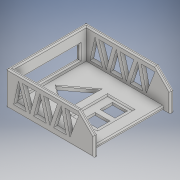
# Autodesk Inventor part: Base-Motherboard-v2
Saved by Autodesk Inventor 2018 (Build 220112000, 112)
## iProperties
Created: 2017-07-20
Part Number: Base-Motherboard-v2
Material: Generic
Document SubType Name: Modeling
Designer: JAck
Density: 1 g/cm^3
Appearance: Default
Author: JAck
Autodesk Inventor part; units mm, degrees
ref_plane "YZ Plane" through (0, 0, 0) normal (1, 0, 0) x (0, 1, 0)
ref_plane "XZ Plane" through (0, 0, 0) normal (0, 1, 0) x (-1, 0, 0)
ref_plane "XY Plane" through (0, 0, 0) normal (0, 0, 1) x (1, 0, 0)
sketch "Sketch1" plane through (0, 0, 0) normal (0, 1, 0) x (-1, 0, 0)
  line L0 (72.6415, 114.85) -> (-102.3585, 114.85)
  line L1 (-102.3585, 114.85) -> (-102.3585, -45.15)
  line L2 (-102.3585, -45.15) -> (72.6415, -45.15)
  line L3 (72.6415, -45.15) -> (72.6415, 114.85)
  line L4 (65.1415, 107.35) -> (-102.3585, 107.35)
  line L5 (-102.3585, 107.35) -> (-102.3585, -37.65)
  line L6 (-102.3585, -37.65) -> (65.1415, -37.65)
  line L7 (65.1415, -37.65) -> (65.1415, 107.35)
  line L8 (-102.3585, -37.65) -> (-89.8585, -37.65)
  line L9 (-89.8585, -37.65) -> (-89.8585, 107.35)
  line L10 (-89.8585, 107.35) -> (-102.3585, 107.35)
  line L11 (-102.3585, 107.35) -> (-102.3585, -37.65)
  point P0 (0, 0)
  dimension "d0" = 175
  dimension "d1" = 160
  dimension "d2" = 7.5
  dimension "d3" = 0
  dimension "d4" = 7.5
  dimension "d5" = 7.5
  dimension "d6" = 145
  dimension "d7" = 167.5
  dimension "d8" = 12.5
  constraints: 24 end point, 6 parallel, 3 horizontal, 3 perpendicular, 1 point on line
  measures "d0" distance between parallel lines of L1 L3
  measures "d1" distance of L0.end L1.end
  measures "d2" distance between parallel lines of L3 L7
  measures "d3" distance between parallel lines of L1 L5
  measures "d4" distance between parallel lines of L2 L6
  measures "d5" distance between parallel lines of L0 L4
  measures "d6" distance between parallel lines of L6 L4
  measures "d7" distance between parallel lines of L5 L7
  measures "d8" distance between parallel lines of L9 L1
extrude "Extrusion1" add sketch "Sketch1" along normal blind 60 contours L3 L2 L1 L6 L7 L4 L0
sketch "Sketch2" plane through (-72.6415, 0, -45.15) normal (-1, 0, 0) x (0, 0, 1)
  line L0 (20, 52.5) -> (140, 52.5)
  line L1 (140, 52.5) -> (140, 25)
  line L2 (140, 25) -> (20, 25)
  line L3 (20, 25) -> (20, 52.5)
  line L4 (160, 0) -> (160, 60) projected
  line L5 (0, 0) -> (0, 60) projected
  line L6 (0, 60) -> (160, 60) projected
  line L7 (0, 0) -> (160, 0) projected
  point P0 (45.15, 0)
  dimension "d11" = 20
  dimension "d12" = 20
  dimension "d13" = 7.5
  dimension "d14" = 25
  dimension "d15" = 120
  dimension "d16" = 27.5
  constraints: 8 end point, 2 parallel, 1 horizontal, 1 perpendicular
  measures "d11" distance between parallel lines of L4 L1
  measures "d12" distance between parallel lines of L5 L3
  measures "d13" distance between parallel lines of L6 L0
  measures "d14" distance between parallel lines of L7 L2
  measures "d15" distance between parallel lines of L3 L1
  measures "d16" distance of L0.end L1.end
extrude "Extrusion2" cut sketch "Sketch2" against normal blind 60 contours L0 L1 L2 L3
sketch "Sketch3" plane through (0, 60, 0) normal (0, 1, 0) x (1, 0, 0)
  line L0 (-72.6415, -114.85) -> (102.3585, -114.85) projected
  line L1 (102.3585, 45.15) -> (-72.6415, 45.15) projected
  line L2 (-72.6415, -114.85) -> (102.3585, -114.85)
  line L3 (102.3585, -114.85) -> (102.3585, 45.15)
  line L4 (102.3585, 45.15) -> (-72.6415, 45.15)
  line L5 (-72.6415, 45.15) -> (-72.6415, -114.85)
  point P0 (0, 0)
  constraints: 8 end point, 2 parallel, 1 horizontal, 1 perpendicular
extrude "Extrusion3" add sketch "Sketch3" along normal blind 7.5
sketch "Sketch4" plane through (0, 60, 0) normal (0, -1, 0) x (1, 0, 0)
  line L0 (-65.1415, 107.35) -> (102.3585, 107.35) projected
  line L1 (102.3585, -37.65) -> (-65.1415, -37.65) projected
  line L2 (102.3585, 107.35) -> (89.8585, 107.35)
  line L3 (89.8585, 107.35) -> (89.8585, -37.65)
  line L4 (89.8585, -37.65) -> (102.3585, -37.65)
  line L5 (102.3585, -37.65) -> (102.3585, 107.35)
  point P0 (0, 0)
  dimension "d21" = 12.5
  constraints: 8 end point, 2 parallel, 1 horizontal, 1 perpendicular, 1 point on line
  measures "d21" distance between parallel lines of L5 L3
extrude "Extrusion4" cut sketch "Sketch4" against normal blind 7.5
chamfer "Chamfer1" distance 30 angle 45 2 edges at (102.3585, 0, 111.1) (102.3585, 0, -41.4)
sketch "Sketch5" plane through (0, 67.5, 0) normal (0, 1, 0) x (1, 0, 0)
  line L0 (59.8585, -4.85) -> (29.8585, -4.85)
  line L1 (29.8585, -4.85) -> (29.8585, -29.85)
  line L2 (29.8585, -29.85) -> (59.8585, -29.85)
  line L3 (59.8585, -29.85) -> (59.8585, -4.85)
  line L4 (59.8585, -64.85) -> (29.8585, -64.85)
  line L5 (29.8585, -64.85) -> (29.8585, -39.85)
  line L6 (29.8585, -39.85) -> (59.8585, -39.85)
  line L7 (59.8585, -39.85) -> (59.8585, -64.85)
  line L8 (89.8585, -107.35) -> (89.8585, 37.65) projected
  line L9 (-72.6415, -114.85) -> (102.3585, -114.85) projected
  line L10 (102.3585, 45.15) -> (-72.6415, 45.15) projected
  point P0 (0, 0)
  dimension "d27" = 30
  dimension "d28" = 30
  dimension "d29" = 10
  dimension "d30" = 50
  dimension "d31" = 50
  dimension "d32" = 25
  dimension "d33" = 30
  dimension "d34" = 30
  constraints: 16 end point, 4 parallel, 2 horizontal, 2 perpendicular, 1 point on line
  measures "d27" distance between parallel lines of L8 L3
  measures "d28" distance between parallel lines of L8 L7
  measures "d29" distance between parallel lines of L6 L2
  measures "d30" distance between parallel lines of L9 L4
  measures "d31" distance between parallel lines of L10 L0
  measures "d32" distance of L0.end L1.end
  measures "d33" distance of L0.start L0.end
  measures "d34" distance between parallel lines of L7 L5
extrude "Extrusion5" cut sketch "Sketch5" against normal blind 7.5
sketch "Sketch6" plane through (0, 60, 0) normal (0, -1, 0) x (1, 0, 0)
  line L0 (64.8585, 69.85) -> (14.8585, 69.85)
  line L1 (14.8585, 69.85) -> (14.8585, -0.15)
  line L2 (14.8585, -0.15) -> (64.8585, -0.15)
  line L3 (64.8585, -0.15) -> (64.8585, 69.85)
  line L4 (59.8585, 64.85) -> (59.8585, 39.85) projected
  line L5 (29.8585, 39.85) -> (29.8585, 64.85) projected
  line L6 (29.8585, 64.85) -> (59.8585, 64.85) projected
  line L7 (59.8585, 4.85) -> (29.8585, 4.85) projected
  point P0 (0, 0)
  dimension "d37" = 5
  dimension "d38" = 15
  dimension "d39" = 5
  dimension "d40" = 5
  constraints: 8 end point, 2 parallel, 1 horizontal, 1 perpendicular
  measures "d37" distance between parallel lines of L3 L4
  measures "d38" distance between parallel lines of L5 L1
  measures "d39" distance between parallel lines of L6 L0
  measures "d40" distance between parallel lines of L2 L7
extrude "Extrusion6" cut sketch "Sketch6" against normal blind 2.5
fillet "Fillet1" radius 2.5 33 edges at (89.8585, 60, 34.85) (102.3585, 48.75, -45.15) (87.3585, 15, -45.15) (102.3585, 48.75, 107.35) (102.3585, 48.75, -37.65) (87.3585, 15, -37.65) (87.3585, 15, 107.35) (87.3585, 15, 114.85) (102.3585, 48.75, 114.85) (3.6085, 0, 107.35) (-0.1415, 0, 114.85) (-0.1415, 0, -45.15) (3.6085, 0, -37.65) (-72.6415, 0, 34.85) (-65.1415, 0, 34.85) (-72.6415, 52.5, 34.85) (-72.6415, 38.75, 94.85) (-72.6415, 25, 34.85) (-72.6415, 38.75, -25.15) (-65.1415, 52.5, 34.85) (-65.1415, 38.75, 94.85) (-65.1415, 25, 34.85) (-65.1415, 38.75, -25.15) (-72.6415, 33.75, 114.85) (-72.6415, 33.75, -45.15) (14.8585, 67.5, 114.85) (-72.6415, 67.5, 34.85) (14.8585, 67.5, -45.15) (89.8585, 67.5, 34.85) (14.8585, 60, 34.85) (39.8585, 60, 69.85) (64.8585, 60, 34.85) (39.8585, 60, -0.15)
sketch "Sketch9" plane through (99.8585, 65, -45.15) normal (0, 0, -1) x (-1, 0, 0)
  line L0 (165, -62.5) -> (165, -5) projected
  line L1 (165, -10) -> (0, -10)
  line L2 (0, 0) -> (0, -33.9645) projected
  line L3 (173.9645, -55) -> (21.0355, -55)
  line L4 (0, -33.9645) -> (28.5355, -62.5) projected
  line L5 (170, -62.5) -> (28.5355, -62.5) projected
  line L6 (0, 0) -> (170, 0) projected
  line L7 (157.5, -10) -> (147.5, -55)
  line L8 (147.5, -55) -> (132.5, -10)
  line L9 (125, -10) -> (140, -55)
  line L10 (125, -10) -> (112.5, -55)
  line L11 (105, -55) -> (117.5, -10)
  line L12 (105, -55) -> (92.5, -10)
  line L13 (97.5, -55) -> (85, -10)
  line L14 (85, -10) -> (70, -55)
  line L15 (62.5, -55) -> (77.5, -10)
  line L16 (62.5, -55) -> (52.5, -10)
  line L17 (45, -10) -> (55, -55)
  line L18 (45, -10) -> (27.5, -55)
  point P0 (99.8585, -65)
  dimension "d48" = 7.5
  dimension "d49" = 10
  dimension "d50" = 7.5
  dimension "d51" = 7.5
  dimension "d52" = 7.5
  dimension "d53" = 7.5
  dimension "d54" = 7.5
  dimension "d55" = 7.5
  dimension "d56" = 27.5
  dimension "d57" = 27.5
  dimension "d58" = 27.5
  dimension "d59" = 25
  dimension "d60" = 25
  dimension "d61" = 25
  dimension "d64" = 7.5
  dimension "d65" = 17.5
  constraints: 24 end point, 5 parallel, 3 point on line, 24 other
  measures "d50" distance of L9.end L7.end
  measures "d51" distance of L9.start L8.end
  measures "d52" distance of L11.start L10.end
  measures "d53" distance of L13.start L11.start
  measures "d54" distance of L15.start L14.end
  measures "d55" distance of L17.end L15.start
  measures "d56" distance of L10.end L9.end
  measures "d57" distance of L14.end L13.start
  measures "d58" distance of L18.end L17.end
  measures "d59" distance of L8.end L7.start
  measures "d60" distance of L12.end L11.end
  measures "d61" distance of L16.end L15.end
  measures "d64" distance from line of L0 L7.start
  measures "d65" distance from line of L0 L7.end
extrude "Extrusion7" cut sketch "Sketch9" against normal through all contours L8 L1 L7 | L3 L10 L9 | L18 L17 L3 | L12 L1 L11 | L16 L1 L15 | L3 L14 L13
sketch "Sketch10" plane through (0, 60, 0) normal (0, -1, 0) x (1, 0, 0)
  line L0 (-2.6415, -2.65) -> (-2.6415, 72.35)
  line L1 (-2.6415, 72.35) -> (-52.6415, 34.85)
  line L2 (-52.6415, 34.85) -> (-2.6415, -2.65)
  line L3 (71.3229, -37.65) -> (-65.1415, -37.65) projected
  line L4 (-65.1415, 107.35) -> (71.3229, 107.35) projected
  line L5 (12.3585, 72.35) -> (12.3585, -2.65) projected
  point P0 (0, 0)
  dimension "d66" = 75
  dimension "d67" = 35
  dimension "d68" = 35
  dimension "d69" = 15
  dimension "d70" = 50
  dimension "d71" = 37.5
  constraints: 6 end point, 1 vertical
  measures "d66" distance of L0.start L0.end
  measures "d67" distance from line of L3 L0.start
  measures "d68" distance from line of L4 L0.end
  measures "d69" distance between parallel lines of L5 L0
  measures "d70" distance from line of L0 L1.end
  measures "d71" vertical distance of L1.end L0.start
extrude "Extrusion8" cut sketch "Sketch10" against normal blind 10
fillet "Fillet2" radius 1.5 3 edges at (-27.6415, 60, 16.1) (-27.6415, 60, 53.6) (-2.6415, 60, 34.85)
equation "\"d5\" = d4"
equation "\"d12\" = d11"
equation "\"d30\" = d31"
equation "\"d34\" = d33"
equation "\"d52\" = d50"
equation "\"d53\" = d50"
equation "\"d54\" = d53"
equation "\"d55\" = d54"
equation "\"d56\" = d57"
equation "\"d58\" = d57"
equation "\"d59\" = d60"
equation "\"d60\" = d61"
equation "\"d71\" = 0.5 * d66"
body "Solid1"
